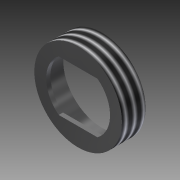
# Autodesk Inventor part: Spring torque cap
Saved by Autodesk Inventor 2012 (Build 160160000, 160)
## iProperties
Created: 2012-06-30
Part Number: Spring torque cap
Material: Default
Document SubType Name: Modeling
Designer: Bruce
Density: 1 g/cm^3
Author: Bruce
Autodesk Inventor part; units mm, degrees
ref_plane "YZ Plane" through (0, 0, 0) normal (1, 0, 0) x (0, 1, 0)
ref_plane "XZ Plane" through (0, 0, 0) normal (0, 1, 0) x (-1, 0, 0)
ref_plane "XY Plane" through (0, 0, 0) normal (0, 0, 1) x (1, 0, 0)
sketch "Sketch1" plane through (0, 0, 0) normal (0, 0, 1) x (1, 0, 0)
  circle A0 centre (0, 0) radius 20.8915
  circle A1 centre (0, 0) radius 15.24
  line L0 (-9.2613, 12.1031) -> (9.2613, 12.1031)
  line L1 (-9.2613, -12.1031) -> (9.2613, -12.1031)
  circle A2 centre (0, 0) radius 18.4404
  dimension "d0" = 41.783
  dimension "d1" = 30.48
  dimension "d2" = 12.1031
  dimension "d3" = 12.1031
  dimension "d4" = 36.8808
  constraints: 4 end point, 4 point on circle, 3 centre point, 3 coincident, 1 horizontal, 1 parallel
  measures "d0" diameter of A0
  measures "d1" diameter of A1
  measures "d2" distance from line of L1 point (0, 0)
  measures "d3" distance from line of L0 point (0, 0)
  measures "d4" diameter of A2
extrude "Extrusion1" add sketch "Sketch1" against normal blind 9.2964 contours A0
extrude "Extrusion2" add sketch "Sketch1" along normal blind 2.032 contours A0 | L0 A1 | A1 L1 | A2
thread "Thread1" size "1 11/16-6 UN" class "2A" standard "ANSI Unified Screw Threads" full length
equation "\"d3\" = d2"
body "Solid1"
